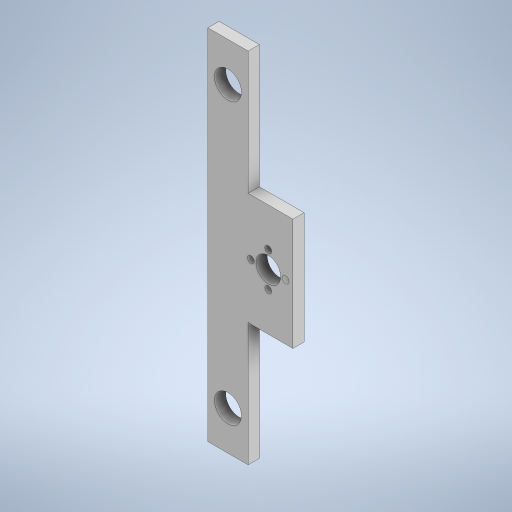
# Autodesk Inventor part: joining brace
Saved by Autodesk Inventor 2023.2 (Build 272271000, 271)
## iProperties
Created: 2023-02-03
Part Number: joining brace
Material: Generic
Document SubType Name: Modeling
Designer: dmargari
Density: 1 g/cm^3
Appearance: Default
Author: dmargari
## iProperties of the stored document joining brace_3DPrint.ipt
Created: 2023-02-03
Part Number: joining brace_3DPrint
Material: Generic
Document SubType Name: Modeling
Designer: dmargari
Density: 1 g/cm^3
Appearance: Default
Author: dmargari
Autodesk Inventor part; units mm, degrees
ref_plane "YZ Plane" through (0, 0, 0) normal (1, 0, 0) x (0, 1, 0)
ref_plane "XZ Plane" through (0, 0, 0) normal (0, 1, 0) x (-1, 0, 0)
ref_plane "XY Plane" through (0, 0, 0) normal (0, 0, 1) x (1, 0, 0)
sketch "Sketch1" plane through (0, 0, 0) normal (0, 0, 1) x (1, 0, 0)
  line L0 (-1.8476, 32.2509) -> (-1.8476, -127.7491)
  line L1 (-1.8476, 32.2509) -> (158.1524, 32.2509) construction
  line L2 (-1.8476, -127.7491) -> (16.1524, -127.7491)
  line L3 (16.1524, -127.7491) -> (16.1524, 32.2509)
  line L4 (16.1524, 32.2509) -> (-1.8476, 32.2509)
  line L5 (7.1524, 32.2509) -> (7.1524, -127.7491) construction
  line L6 (-1.8476, -47.7491) -> (16.1524, -47.7491) construction
  circle A0 centre (7.1524, -110.3056) radius 6
  circle A1 centre (7.1524, 14.8074) radius 6
  line L7 (16.1524, -22.7491) -> (36.1524, -22.7491)
  line L8 (36.1524, -22.7491) -> (36.1524, -72.7491)
  line L9 (36.1524, -72.7491) -> (16.1524, -72.7491)
  line L10 (16.1524, -47.7491) -> (36.1524, -47.7491) construction
  circle A2 centre (25.1524, -47.7491) radius 5.5
  point P0 (0, 0)
  dimension "d0" = 160
  dimension "d1" = 90
  dimension "d2" = 18
  dimension "d3" = 12
  dimension "d4" = 12
  dimension "d5" = 125.113
  dimension "d6" = 20
  dimension "d7" = 50
  dimension "d8" = 55
  dimension "d15" = 11
  dimension "d16" = 9
  dimension "d17" = 17.4435
  dimension "d25" = 9
  constraints: 22 end point, 5 midpoint, 5 perpendicular, 5 point on line, 3 centre point, 2 horizontal, 2 vertical
  measures "d0" distance of L0.start L0.end
  measures "d1" angle of L0 L1
  measures "d2" distance of L0.end L2.end
  measures "d3" diameter of A0
  measures "d4" diameter of A1
  measures "d5" distance of A1.centre A0.centre
  measures "d6" distance of L7.start L7.end
  measures "d7" distance of L7.end L8.end
  measures "d8" distance between parallel lines of L1 L7
  measures "d15" diameter of A2
  measures "d16" distance from line of A2.centre L3
  measures "d17" distance from line of A1.centre L4
  measures "d25" distance between parallel lines of L0 L5
extrude "Extrusion1" add sketch "Sketch1" along normal blind 5
sketch "Sketch2" plane through (0, 0, 0) normal (0, 0, 1) x (1, 0, 0)
  circle A0 centre (25.1524, -55.4991) radius 1.5 projected
  circle A1 centre (17.4024, -47.7491) radius 1.5 projected
  circle A2 centre (25.1524, -39.9991) radius 1.5 projected
  circle A3 centre (32.9024, -47.7491) radius 1.5 projected
  point P0 (0, 0)
hole "Hole1" at (25.1524, -55.4991, 0) at (32.9024, -47.7491, 0) at (25.1524, -39.9991, 0) at (17.4024, -47.7491, 0) direction (0, 0, 1) diameter 3 end through all
equation "\"d8\" = 0.5 * d0 - 0.5 * d7"
equation "\"d17\" = 0.5 * d0 - 0.5 * d5"
body "Solid1"
